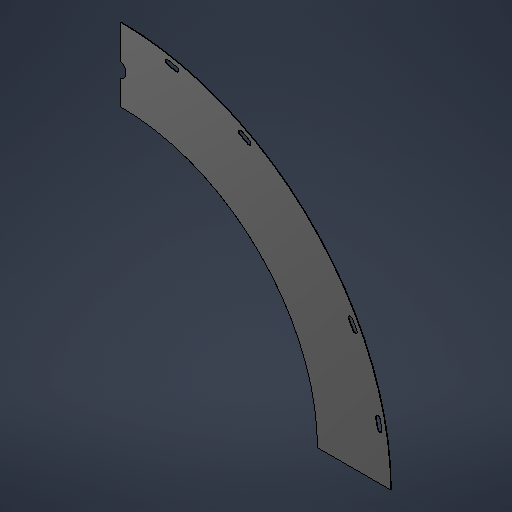
# Autodesk Inventor part: 3DPRINT,CABLE,TRAY
Saved by Autodesk Inventor 2026.1 (Build 301233020, 233B)
## iProperties
Created: 2026-02-14
Part Number: 3DPRINT,CABLE,TRAY
Material: ABS Plastic
Document SubType Name: Modeling
Designer: Owen L
Density: 1.06 g/cm^3
Appearance: Smooth - Black
Author: Owen L
Autodesk Inventor part; units mm, degrees
ref_plane "YZ Plane" through (0, 0, 0) normal (1, 0, 0) x (0, 1, 0)
ref_plane "XZ Plane" through (0, 0, 0) normal (0, 1, 0) x (-1, 0, 0)
ref_plane "XY Plane" through (0, 0, 0) normal (0, 0, 1) x (1, 0, 0)
sketch "Sketch1" plane through (0, 0, 0) normal (0, 0, 1) x (1, 0, 0)
  arc A0 (187.325, 0) -> (0, 187.325) centre (0, 0) ccw
  arc A1 (136.525, 0) -> (0, 136.525) centre (0, 0) ccw
  line L0 (0, 136.525) -> (0, 187.325)
  line L1 (136.525, 0) -> (187.325, 0)
  point P0 (161.925, 0)
  point P1 (0, 161.925)
  dimension "d2" = 187.325
  dimension "d3" = 136.525
  constraints: 4 end point, 4 point on circle, 2 centre point, 2 coincident, 2 midpoint, 1 horizontal alignment, 1 perpendicular, 1 vertical, 1 vertical alignment
  measures "d2" radius of A0
  measures "d3" radius of A1
extrude "Extrusion1" add sketch "Sketch1" along normal blind 0.4
sketch "Sketch3" plane through (0, 0, 0.4) normal (0, 0, 1) x (1, 0, 0)
  arc A0 (178.117, 32.1925) -> (181.231, 32.8119) centre (179.674, 32.5022) ccw projected
  line L0 (178.117, 32.1925) -> (176.8782, 38.4205) projected
  arc A1 (179.9922, 39.0399) -> (176.8782, 38.4205) centre (178.4352, 38.7302) ccw projected
  line L1 (179.9922, 39.0399) -> (181.231, 32.8119) projected
  line L2 (160.9091, 89.6078) -> (163.9025, 84.0076) projected
  arc A2 (161.1024, 82.5109) -> (163.9025, 84.0076) centre (162.5024, 83.2593) ccw projected
  line L3 (161.1024, 82.5109) -> (158.109, 88.1111) projected
  arc A3 (160.9091, 89.6078) -> (158.109, 88.1111) centre (159.5091, 88.8595) ccw projected
  line L4 (84.0076, 163.9025) -> (89.6078, 160.9091) projected
  arc A4 (84.0076, 163.9025) -> (82.5109, 161.1024) centre (83.2593, 162.5024) ccw projected
  line L5 (88.1111, 158.109) -> (82.5109, 161.1024) projected
  arc A5 (88.1111, 158.109) -> (89.6078, 160.9091) centre (88.8595, 159.5091) ccw projected
  arc A6 (38.4205, 176.8782) -> (39.0399, 179.9922) centre (38.7302, 178.4352) ccw projected
  line L6 (32.8119, 181.231) -> (39.0399, 179.9922) projected
  arc A7 (32.8119, 181.231) -> (32.1925, 178.117) centre (32.5022, 179.674) ccw projected
  line L7 (38.4205, 176.8782) -> (32.1925, 178.117) projected
  circle A8 centre (-1.6445, 158.6401) radius 5.334 projected
  point P0 (0, 0)
extrude "Extrusion2" cut sketch "Sketch3" against normal through all
body "Solid1"
